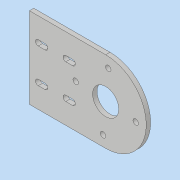
# Autodesk Inventor part: MMplate2
Saved by Autodesk Inventor 2017 (Build 210142000, 142)
## iProperties
Created: 2016-12-23
Part Number: MMplate2
Material: Generic
Document SubType Name: Modeling
Designer: Joshua Yuan
Density: 1 g/cm^3
Appearance: Default
Author: Joshua Yuan
Autodesk Inventor part; units mm, degrees
ref_plane "YZ Plane" through (0, 0, 0) normal (1, 0, 0) x (0, 1, 0)
ref_plane "XZ Plane" through (0, 0, 0) normal (0, 1, 0) x (-1, 0, 0)
ref_plane "XY Plane" through (0, 0, 0) normal (0, 0, 1) x (1, 0, 0)
sketch "Sketch1" plane through (0, 0, 0) normal (0, 0, 1) x (1, 0, 0)
  circle A0 centre (187.7995, 54.1889) radius 29.5
  line L0 (187.7995, 83.6889) -> (132.2995, 83.6889)
  line L1 (132.2995, 83.6889) -> (132.2995, 24.6889)
  line L2 (132.2995, 24.6889) -> (187.7995, 24.6889)
  circle A1 centre (187.7995, 54.1889) radius 9.525
  circle A2 centre (165.9626, 56.0994) radius 2
  circle A3 centre (189.7099, 76.0258) radius 2
  circle A4 centre (209.6364, 52.2784) radius 2
  circle A5 centre (185.889, 32.352) radius 2
  line L3 (189.7099, 76.0258) -> (185.889, 32.352) construction
  line L4 (209.6364, 52.2784) -> (165.9626, 56.0994) construction
  line L5 (-43.4599, 0) -> (260.7594, 0) projected
  line L6 (0, -16.7378) -> (0, 100.4267) projected
  line L7 (187.7995, 54.1889) -> (120.7595, 54.1889) construction
  circle A6 centre (138.7402, 66.6889) radius 2.0193
  circle A7 centre (143.7402, 66.6889) radius 2.0193
  circle A8 centre (158.7411, 66.7517) radius 2.0193
  circle A9 centre (163.7411, 66.7517) radius 2.0193
  circle A10 centre (143.7402, 41.6889) radius 2.0193
  circle A11 centre (138.7402, 41.6889) radius 2.0193
  circle A12 centre (163.7402, 41.6889) radius 2.0193
  circle A13 centre (158.7402, 41.6889) radius 2.0193
  line L8 (143.7402, 68.7082) -> (138.7402, 68.7082)
  line L9 (138.7402, 64.6696) -> (143.7402, 64.6696)
  line L10 (158.7411, 68.771) -> (163.7411, 68.771)
  line L11 (163.7411, 64.7324) -> (158.7411, 64.7324)
  line L12 (163.7402, 43.7082) -> (158.7402, 43.7082)
  line L13 (158.7402, 39.6696) -> (163.7402, 39.6696)
  line L14 (143.7402, 43.7082) -> (138.7402, 43.7082)
  line L15 (138.7402, 39.6696) -> (143.7402, 39.6696)
  circle A14 centre (140.7595, 66.6889) radius 2.0193 construction
  circle A15 centre (140.7595, 41.6889) radius 2.0193 construction
  line L16 (140.7595, 66.6889) -> (140.7595, 41.6889) construction
  circle A16 centre (160.7595, 41.6889) radius 2.0193 construction
  circle A17 centre (160.7595, 66.6889) radius 2.0193 construction
  line L17 (160.7595, 66.6889) -> (160.7595, 41.6889) construction
  point P0 (0, 0)
  dimension "d26" = 4.0386
  dimension "d0" = 59
  dimension "d1" = 55.5
  dimension "d2" = 19.05
  dimension "d3" = 4
  dimension "d4" = 4
  dimension "d5" = 4
  dimension "d6" = 4
  dimension "d7" = 355
  dimension "d8" = 31
  dimension "d9" = 31
  dimension "d10" = 31
  dimension "d11" = 67.04
  dimension "d13" = 4.0386
  dimension "d14" = 4.0386
  dimension "d16" = 4.0386
  dimension "d17" = 4.0386
  dimension "d18" = 4.0386
  dimension "d19" = 4.0386
  dimension "d20" = 4.0386
  dimension "d21" = 4.0386
  dimension "d22" = 5
  dimension "d23" = 5
  dimension "d24" = 5
  dimension "d25" = 5
  dimension "d27" = 20
  dimension "d29" = 20
  dimension "d32" = 25
  constraints: 32 end point, 21 point on circle, 20 tangent, 15 centre point, 7 horizontal, 4 symmetric about line, 3 perpendicular, 2 coincident, 2 equal length, 2 horizontal alignment, 2 midpoint, 2 vertical, 1 parallel, 7 other
  measures "d0" diameter of A0
  measures "d1" distance of L0.start L0.end
  measures "d2" diameter of A1
  measures "d3" diameter of A2
  measures "d4" diameter of A3
  measures "d5" diameter of A4
  measures "d6" diameter of A5
  measures "d8" distance of L3.end L4.start
  measures "d9" distance of L4.end L3.end
  measures "d10" distance of L3.start L4.start
  measures "d11" distance of L7.start L7.end
  measures "d13" diameter of A6
  measures "d14" diameter of A7
  measures "d16" diameter of A8
  measures "d17" diameter of A9
  measures "d18" diameter of A10
  measures "d19" diameter of A11
  measures "d20" diameter of A12
  measures "d21" diameter of A13
  measures "d22" distance of A6.centre A7.centre
  measures "d23" distance of A9.centre A8.centre
  measures "d24" distance of A12.centre A13.centre
  measures "d25" distance of A11.centre A10.centre
  measures "d27" distance from line of point (120.759, 54.189) L16
  measures "d29" distance between parallel lines of L17 L16
  measures "d32" distance of L16.start L16.end
extrude "Extrusion1" add sketch "Sketch1" along normal blind 3.175 contours A0 L13 A12 L12 L11 A9 L10 | A0 L10 A8 L11 L12 A13 L13 L2 L1 L0
body "Solid1"
